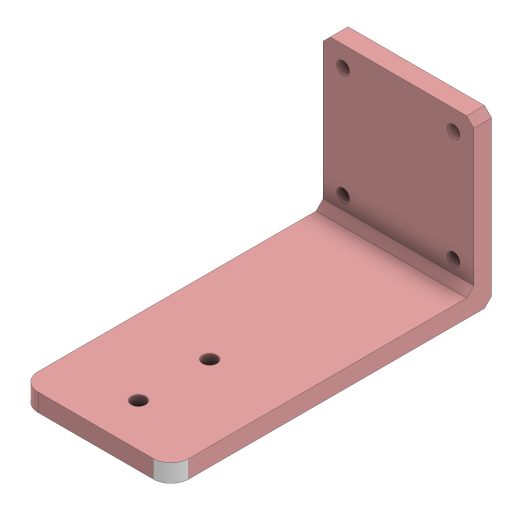
# Autodesk Inventor part: ACOPLE PARA NEMA DE CAJA
Saved by Autodesk Inventor 2024 (Build 280153000, 153)
## iProperties
Created: 2024-07-10
Part Number: ACOPLE PARA NEMA DE CAJA
Material: Generic
Document SubType Name: Modeling
Designer: Jhuliams
Density: 1 g/cm^3
Appearance: Default
Author: Jhuliams
Autodesk Inventor part; units mm, degrees
ref_plane "YZ Plane" through (0, 0, 0) normal (1, 0, 0) x (0, 1, 0)
ref_plane "XZ Plane" through (0, 0, 0) normal (0, 1, 0) x (-1, 0, 0)
ref_plane "XY Plane" through (0, 0, 0) normal (0, 0, 1) x (1, 0, 0)
sketch "Sketch1" plane through (0, 0, 0) normal (0, 1, 0) x (-1, 0, 0)
  line L0 (21.15, 45) -> (-21.15, 45)
  line L1 (-21.15, 45) -> (-21.15, -45)
  line L2 (-21.15, -45) -> (21.15, -45)
  line L3 (21.15, -45) -> (21.15, 45)
  line L4 (21.15, 45) -> (-21.15, -45) construction
  line L5 (-21.15, 45) -> (21.15, -45) construction
  point P0 (0, 0)
  dimension "d0" = 42.3
  dimension "d1" = 90
  constraints: 12 end point, 2 midpoint, 2 parallel, 1 horizontal, 1 perpendicular
  measures "d0" distance of L2.end L1.end
  measures "d1" distance of L1.end L0.end
extrude "Extrusion1" add sketch "Sketch1" along normal blind 5
sketch "Sketch2" plane through (0, 5, 0) normal (0, 1, 0) x (1, 0, 0)
  line L0 (0, 0) -> (0, 42.5)
  line L1 (21.15, -45) -> (21.15, 45) projected
  line L2 (-21.15, 40) -> (21.15, 40)
  line L3 (21.15, 40) -> (21.15, 45)
  line L4 (21.15, 45) -> (-21.15, 45)
  line L5 (-21.15, 45) -> (-21.15, 40)
  line L6 (-21.15, 40) -> (21.15, 45) construction
  line L7 (21.15, 40) -> (-21.15, 45) construction
  dimension "d4" = 42.5
  dimension "d5" = 42.3
  dimension "d6" = 5
  constraints: 14 end point, 2 midpoint, 2 parallel, 1 horizontal, 1 perpendicular, 1 vertical
  measures "d4" distance of L0.start L0.end
  measures "d5" distance of L4.end L1.end
  measures "d6" distance of L1.end L2.end
extrude "Extrusion2" add sketch "Sketch2" along normal blind 42.3
sketch "Sketch3" plane through (-21.15, 5, -40) normal (0, 0, 1) x (1, 0, 0)
  line L0 (42.3, 0) -> (0, 0) projected
  line L1 (42.3, 0) -> (42.3, 42.3) projected
  line L2 (0, 42.3) -> (42.3, 42.3) projected
  line L3 (0, 0) -> (0, 42.3) projected
  line L4 (42.3, 42.3) -> (0, 0)
  line L5 (5.65, 36.65) -> (36.65, 36.65)
  line L6 (36.65, 36.65) -> (36.65, 5.65)
  line L7 (36.65, 5.65) -> (5.65, 5.65)
  line L8 (5.65, 5.65) -> (5.65, 36.65)
  line L9 (5.65, 36.65) -> (36.65, 5.65) construction
  line L10 (36.65, 36.65) -> (5.65, 5.65) construction
  circle A0 centre (5.65, 36.65) radius 1.75
  circle A1 centre (36.65, 36.65) radius 1.75
  circle A2 centre (5.65, 5.65) radius 1.75
  circle A3 centre (36.65, 5.65) radius 1.75
  point P0 (21.15, -5)
  point P1 (21.15, 21.15)
  dimension "d9" = 31
  dimension "d10" = 31
  dimension "d11" = 3.5
  dimension "d14" = 31
  dimension "d17" = 31
  constraints: 14 end point, 4 centre point, 3 midpoint, 2 horizontal, 2 parallel, 1 coincident, 1 perpendicular, 1 vertical, 6 other
  measures "d9" distance of L6.end L7.end
  measures "d10" distance of L5.end L6.end
  measures "d11" diameter of A0
  measures "d14" distance of A0.centre A1.centre
  measures "d17" distance of A0.centre A2.centre
extrude "Extrusion3" cut sketch "Sketch3" against normal blind 42.3 contours A2 L8 L4 | L4 L7 A2 | A1 L6 L4 | L4 L5 A1 | L8 A2 L4 | L4 A2 L7 | L6 A1 L4 | L4 A1 L5 | A0 L5 L8 | L8 L5 A0 | A3 L6 L7 | L7 L6 A3
chamfer "Chamfer1" distance 2 angle 45 1 edges at (0, 5, -40)
chamfer "Chamfer2" distance 2 angle 45 3 edges at (21.15, 47.3, -42.5) (-21.15, 47.3, -42.5) (0, 0, -45)
sketch "Sketch4" plane through (0, 5, 0) normal (0, 1, 0) x (1, 0, 0)
  line L0 (-21.15, -45) -> (21.15, -45) projected
  line L1 (0, -45) -> (0, -33)
  line L2 (0, -33) -> (0, -13)
  circle A0 centre (0, -33) radius 2
  circle A1 centre (0, -13) radius 2
  point P0 (0, 0)
  dimension "d28" = 12
  dimension "d29" = 20
  dimension "d30" = 4
  dimension "d31" = 4
  constraints: 4 end point, 2 centre point, 2 coincident, 1 midpoint, 1 point on line, 1 vertical
  measures "d28" distance of L1.start L1.end
  measures "d29" distance of L1.end L2.end
  measures "d30" diameter of A0
  measures "d31" diameter of A1
sketch "Sketch5" plane through (21.15, 2, -45) normal (0, 0, -1) x (-1, 0, 0)
  circle A0 centre (5.65, 39.65) radius 1.75 projected
  circle A1 centre (36.65, 39.65) radius 1.75 projected
  circle A2 centre (5.65, 8.65) radius 1.75 projected
  circle A3 centre (36.65, 8.65) radius 1.75 projected
  circle A4 centre (5.65, 39.65) radius 2.5
  circle A5 centre (36.65, 39.65) radius 2.5
  circle A6 centre (5.65, 8.65) radius 2.5
  circle A7 centre (36.65, 8.65) radius 2.5
  point P0 (21.15, -2)
  dimension "d32" = 5
  dimension "d33" = 5
  dimension "d34" = 5
  dimension "d35" = 5
  constraints: 4 centre point, 4 coincident
  measures "d32" diameter of A4
  measures "d33" diameter of A5
  measures "d34" diameter of A6
  measures "d35" diameter of A7
extrude "Extrusion4" cut sketch "Sketch5" against normal blind 2 contours A0 | A1 | A2 | A3 | A4 | A5 | A6 | A7
extrude "Extrusion5" cut sketch "Sketch4" against normal blind 5
fillet "Fillet1" radius 5 2 edges at (21.15, 2.5, 45) (-21.15, 2.5, 45)
body "Solid1"
